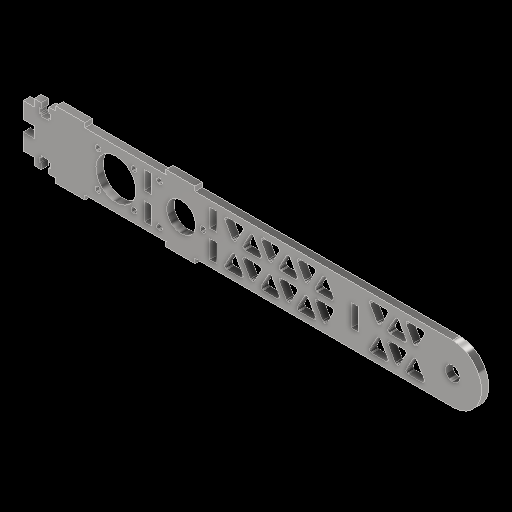
# Autodesk Inventor part: NeckFrame_Draft04
Saved by Autodesk Inventor 2022 (Build 260153000, 153)
## iProperties
Created: 2021-03-08
Part Number: NeckFrame_Draft04
Material: Steel, High Strength, Low Alloy
Document SubType Name: Modeling
Designer: M3rob
Density: 7.85 g/cm^3
Appearance: Steel - Polished
Mass: 5825.21 g
Surface Area: 1820.51 cm^2
Volume: 742.065 cm^3
Author: M3rob
Autodesk Inventor part; units mm, degrees
ref_plane "YZ Plane" through (0, 0, 0) normal (1, 0, 0) x (0, 1, 0)
ref_plane "XZ Plane" through (0, 0, 0) normal (0, 1, 0) x (-1, 0, 0)
ref_plane "XY Plane" through (0, 0, 0) normal (0, 0, 1) x (1, 0, 0)
sketch "Sketch1" plane through (0, 0, 0) normal (1, 0, 0) x (0, 1, 0)
  line L0 (50.8, 392.0089) -> (38.1, 392.0089)
  line L1 (-50.8, 392.0089) -> (-50.8, 366.2152)
  arc A0 (-50.8, -341.2089) -> (50.8, -341.2089) centre (0, -341.2089) ccw
  line L2 (50.8, -341.2089) -> (50.8, 110.0689)
  line L3 (50.8, -341.2089) -> (50.8, -392.0089) construction
  line L4 (50.8, -392.0089) -> (-50.8, -392.0089) construction
  line L5 (-50.8, -392.0089) -> (-50.8, -341.2089) construction
  line L6 (0, 392.0089) -> (0, -392.0089) construction
  line L7 (38.1, 392.0089) -> (38.1, 411.0589)
  line L8 (38.1, 411.0589) -> (9.525, 411.0589)
  line L9 (9.525, 411.0589) -> (9.525, 392.0089)
  line L10 (-9.525, 392.0089) -> (-9.525, 411.0589)
  line L11 (-9.525, 411.0589) -> (-38.1, 411.0589)
  line L12 (-38.1, 411.0589) -> (-38.1, 392.0089)
  line L13 (9.525, 392.0089) -> (-9.525, 392.0089)
  line L14 (38.1, 392.0089) -> (9.525, 392.0089) construction
  line L15 (-9.525, 392.0089) -> (-38.1, 392.0089) construction
  line L16 (-38.1, 392.0089) -> (-50.8, 392.0089)
  line L17 (39.6875, 84.6689) -> (7.9375, 84.6689)
  line L18 (7.9375, 84.6689) -> (7.9375, 71.9689)
  line L19 (7.9375, 71.9689) -> (39.6875, 71.9689)
  line L20 (39.6875, 71.9689) -> (39.6875, 84.6689)
  line L21 (39.6875, 84.6689) -> (7.9375, 71.9689) construction
  line L22 (7.9375, 84.6689) -> (39.6875, 71.9689) construction
  line L23 (-39.6875, 84.6689) -> (-7.9375, 84.6689)
  line L24 (-7.9375, 84.6689) -> (-7.9375, 71.9689)
  line L25 (-7.9375, 71.9689) -> (-39.6875, 71.9689)
  line L26 (-39.6875, 71.9689) -> (-39.6875, 84.6689)
  line L27 (-39.6875, 84.6689) -> (-7.9375, 71.9689) construction
  line L28 (-7.9375, 84.6689) -> (-39.6875, 71.9689) construction
  line L29 (50.8, 353.9089) -> (58.7375, 353.9089)
  line L30 (58.7375, 353.9089) -> (58.7375, 303.1089)
  line L31 (58.7375, 303.1089) -> (50.8, 303.1089)
  line L32 (50.8, 160.8689) -> (58.7375, 160.8689)
  line L33 (58.7375, 160.8689) -> (58.7375, 110.0689)
  line L34 (58.7375, 110.0689) -> (50.8, 110.0689)
  line L35 (-50.8, 110.0689) -> (-58.7375, 110.0689)
  line L36 (-58.7375, 110.0689) -> (-58.7375, 160.8689)
  line L37 (-58.7375, 160.8689) -> (-50.8, 160.8689)
  line L38 (7.9375, 198.9689) -> (39.6875, 198.9689)
  line L39 (39.6875, 198.9689) -> (39.6875, 186.2689)
  line L40 (39.6875, 186.2689) -> (7.9375, 186.2689)
  line L41 (7.9375, 186.2689) -> (7.9375, 198.9689)
  line L42 (7.9375, 198.9689) -> (39.6875, 186.2689) construction
  line L43 (39.6875, 198.9689) -> (7.9375, 186.2689) construction
  line L44 (-39.6875, 198.9689) -> (-7.9375, 198.9689)
  line L45 (-7.9375, 198.9689) -> (-7.9375, 186.2689)
  line L46 (-7.9375, 186.2689) -> (-39.6875, 186.2689)
  line L47 (-39.6875, 186.2689) -> (-39.6875, 198.9689)
  line L48 (-39.6875, 198.9689) -> (-7.9375, 186.2689) construction
  line L49 (-7.9375, 198.9689) -> (-39.6875, 186.2689) construction
  line L50 (23.8125, 192.6189) -> (23.8125, 78.3189) construction
  line L51 (-50.8, 353.9089) -> (-58.7375, 353.9089)
  line L52 (-58.7375, 353.9089) -> (-58.7375, 303.1089)
  line L53 (-58.7375, 303.1089) -> (-50.8, 303.1089)
  line L54 (50.8, 303.1089) -> (50.8, 353.9089) construction
  line L55 (50.8, 353.9089) -> (50.8, 392.0089) construction
  line L56 (-50.8, 303.1089) -> (-50.8, 353.9089) construction
  line L57 (-50.8, 353.9089) -> (-50.8, 303.1089) construction
  line L58 (-50.8, 160.8689) -> (-50.8, 110.0689) construction
  line L59 (-50.8, 110.0689) -> (-50.8, -341.2089)
  line L60 (50.8, 160.8689) -> (50.8, 303.1089)
  line L61 (50.8, 110.0689) -> (50.8, 160.8689) construction
  line L62 (50.8, 379.7026) -> (41.275, 379.7026)
  line L63 (41.275, 379.7026) -> (41.275, 382.4839)
  line L64 (41.275, 382.4839) -> (33.3375, 382.4839)
  line L65 (33.3375, 382.4839) -> (33.3375, 379.7026)
  line L66 (33.3375, 379.7026) -> (30.1625, 379.7026)
  line L67 (30.1625, 379.7026) -> (30.1625, 366.2152)
  line L68 (30.1625, 366.2152) -> (33.3375, 366.2152)
  line L69 (33.3375, 366.2152) -> (33.3375, 363.4339)
  line L70 (33.3375, 363.4339) -> (41.275, 363.4339)
  line L71 (41.275, 363.4339) -> (41.275, 366.2152)
  line L72 (41.275, 366.2152) -> (50.8, 366.2152)
  line L73 (30.1625, 372.9589) -> (50.8, 372.9589) construction
  line L74 (-50.8, 379.7026) -> (-41.275, 379.7026)
  line L75 (-41.275, 379.7026) -> (-41.275, 382.4839)
  line L76 (-41.275, 382.4839) -> (-33.3375, 382.4839)
  line L77 (-33.3375, 382.4839) -> (-33.3375, 379.7026)
  line L78 (-33.3375, 379.7026) -> (-30.1625, 379.7026)
  line L79 (-30.1625, 379.7026) -> (-30.1625, 366.2152)
  line L80 (-30.1625, 366.2152) -> (-33.3375, 366.2152)
  line L81 (-33.3375, 366.2152) -> (-33.3375, 363.4339)
  line L82 (-33.3375, 363.4339) -> (-41.275, 363.4339)
  line L83 (-41.275, 363.4339) -> (-41.275, 366.2152)
  line L84 (-50.8, 366.2152) -> (-41.275, 366.2152)
  line L85 (50.8, 379.7026) -> (50.8, 303.1089) construction
  line L86 (50.8, 366.2152) -> (50.8, 379.7026)
  line L87 (-50.8, 366.2152) -> (-50.8, 353.9089)
  line L88 (-50.8, 379.7026) -> (-50.8, 366.2152) construction
  circle A1 centre (0, 248.4989) radius 35.179
  circle A2 centre (0, 134.1989) radius 25.4
  line L89 (50.8, 379.7026) -> (50.8, 392.0089)
  line L90 (50.8, 366.2152) -> (50.8, 353.9089)
  circle A3 centre (0, -341.2089) radius 12.7
  line L91 (50.8, 353.9089) -> (50.8, 366.2152)
  line L92 (50.8, 303.1089) -> (50.8, 353.9089)
  line L93 (-50.8, 353.9089) -> (-50.8, 379.7026)
  line L94 (-50.8, 303.1089) -> (-50.8, 160.8689)
  line L95 (-50.8, 353.9089) -> (-50.8, 303.1089) construction
  line L96 (-50.8, 366.2152) -> (-50.8, 353.9089)
  circle A4 centre (0, 248.4989) radius 44.45 construction
  circle A5 centre (31.4309, 279.9298) radius 5.08 construction
  line L97 (31.4309, 279.9298) -> (0, 248.4989) construction
  circle A6 centre (-31.4309, 279.9298) radius 5.08 construction
  circle A7 centre (-31.4309, 217.068) radius 5.08 construction
  circle A8 centre (31.4309, 217.068) radius 5.08 construction
  circle A9 centre (34.925, 172.2989) radius 5.08 construction
  circle A10 centre (-34.925, 172.2989) radius 5.08 construction
  circle A11 centre (0, 96.0989) radius 5.08 construction
  line L98 (19.05, -163.6161) -> (-19.05, -163.6161)
  line L99 (-19.05, -163.6161) -> (-19.05, -176.3161)
  line L100 (-19.05, -176.3161) -> (19.05, -176.3161)
  line L101 (19.05, -176.3161) -> (19.05, -163.6161)
  point P0 (0, 0)
  point P1 (-23.8125, 78.3189)
  point P2 (23.8125, 192.6189)
  point P3 (-23.8125, 192.6189)
  point P4 (23.8125, 411.0589)
  point P5 (58.7375, 135.4689)
  point P6 (23.8125, 135.4689)
  point P7 (23.8125, 372.9589)
  point P8 (-30.1625, 372.9589)
  point P9 (50.8, 353.9089)
  point P10 (50.8, 303.1089)
  point P11 (-50.8, 379.7026)
  point P12 (-50.8, 366.2152)
  point P13 (-50.8, 353.9089)
  point P14 (-50.8, 353.9089)
  point P15 (-50.8, 303.1089)
  point P16 (0, -378.889)
  point P17 (0, 0)
  point P18 (0, -163.6161)
  dimension "d130" = 88.9
  dimension "d0" = 101.6
  dimension "d3" = 19.05
  dimension "d4" = 12.7
  dimension "d5" = 19.05
  dimension "d6" = 12.7
  dimension "d8" = 7.9375
  dimension "d9" = 50.8
  dimension "d12" = 31.75
  dimension "d13" = 38.1
  dimension "d14" = 9.525
  dimension "d15" = 7.9375
  dimension "d16" = 3.175
  dimension "d17" = 19.05
  dimension "d18" = 13.4874
  dimension "d23" = 143.51
  dimension "d24" = 70.358
  dimension "d25" = 50.8
  dimension "d26" = 19.05
  dimension "d39" = 25.4
  dimension "d86" = 101.6
  dimension "d92" = 193.04
  dimension "d98" = 7.9375
  dimension "d99" = 0
  dimension "d100" = 7.9375
  dimension "d101" = 50.8
  dimension "d102" = 34.925
  dimension "d104" = 732.7979
  dimension "d105" = 109.5375
  dimension "d106" = 25.7937
  dimension "d107" = 109.5375
  dimension "d108" = 12.3063
  dimension "d109" = 109.5375
  dimension "d110" = 0
  dimension "d111" = 109.5375
  dimension "d112" = 0
  dimension "d113" = 109.5375
  dimension "d114" = 50.8
  dimension "d116" = 45
  dimension "d118" = 10.16
  dimension "d121" = 360
  dimension "d131" = 114.3
  dimension "d132" = 475.4078
  dimension "d135" = 10.16
  dimension "d136" = 38.1
  dimension "d138" = 38.1
  dimension "d139" = 69.85
  dimension "d161" = 555.625
  dimension "d162" = 12.7
  dimension "d163" = 38.1
  constraints: 204 end point, 125 perpendicular, 34 point on line, 21 tangent, 19 midpoint, 15 equal length, 15 horizontal, 14 vertical, 11 centre point, 11 parallel, 6 horizontal alignment, 3 collinear, 3 vertical alignment, 2 coincident, 2 equal radius, 2 point on circle, 1 concentric, 1 symmetric about line, 18 other
  measures "d0" distance of L0.start L1.start
  measures "d3" diameter of L9 L6
  measures "d4" distance from line of L0.start L7
  measures "d5" distance of L0.end L7.end
  measures "d6" distance of L19.end L17.start
  measures "d8" distance of L33.end L2.end
  measures "d9" distance of L32.end L33.end
  measures "d12" distance of L18.end L19.end
  measures "d13" distance from line of L29 L0.start
  measures "d14" distance of L71.end L72.end
  measures "d15" distance of L69.end L70.end
  measures "d16" distance of L67.end L68.end
  measures "d17" distance of L69.end L64.end
  measures "d18" distance between parallel lines of L72 L62
  measures "d23" distance from line of L14 A1.centre
  measures "d24" diameter of A1
  measures "d25" diameter of A2
  measures "d26" distance from line of L0 L73.end
  measures "d39" diameter of A3
  measures "d86" distance between parallel lines of L40 L17
  measures "d92" distance between parallel lines of L38 L0
  measures "d98" distance from line of point (50.8, 353.909) L30
  measures "d99" distance from line of point (50.8, 353.909) L29
  measures "d100" distance from line of point (50.8, 303.109) L30
  measures "d101" distance from line of point (50.8, 303.109) L29
  measures "d102" distance from line of point (23.812, 372.959) L30
  measures "d104" distance from line of point (0, -378.889) L29
  measures "d105" distance from line of point (-50.8, 379.703) L30
  measures "d106" distance from line of point (-50.8, 379.703) L29
  measures "d107" distance from line of point (-50.8, 366.215) L30
  measures "d108" distance from line of point (-50.8, 366.215) L29
  measures "d109" distance from line of point (-50.8, 353.909) L30
  measures "d110" distance from line of point (-50.8, 353.909) L29
  measures "d111" distance from line of point (-50.8, 353.909) L30
  measures "d112" distance from line of point (-50.8, 353.909) L29
  measures "d113" distance from line of point (-50.8, 303.109) L30
  measures "d114" distance from line of point (-50.8, 303.109) L29
  measures "d116" angle of L6 L97
  measures "d118" diameter of A5
  measures "d131" distance of A2.centre A1.centre
  measures "d132" distance of A0.centre A2.centre
  measures "d135" diameter of A9
  measures "d136" vertical distance of A2.centre A9.centre
  measures "d138" distance of A11.centre A2.centre
  measures "d139" diameter of A9.centre L6
  measures "d161" distance between parallel lines of L98 L13
  measures "d162" distance between parallel lines of L100 L98
  measures "d163" distance of L98.start L98.end
extrude "Extrusion1" add sketch "Sketch1" along normal mid plane 12.7 contours L89 L62 L63 L64 L65 L66 L67 L68 L69 L70 L71 L72 L90 L92 L60 L32 L33 L34 L2 A0 L59 L35 L36 L37 L94 L53 L52 L51 L87 L84 L83 L82 L81 L80 L79 L78 L77 L76 L75 L74 L1 L16 L12 L11 L10 L13 L9 L8 L7 L0 | L29 L30 L31 L92
sketch "Sketch6" plane through (6.35, 0, 0) normal (1, 0, 0) x (0, 0, -1)
  point P0 (0, 0)
  point P1 (-279.9298, 31.4309)
  point P2 (-279.9298, -31.4309)
  point P3 (-217.068, -31.4309)
  point P4 (-217.068, 31.4309)
  point P5 (-172.2989, 34.925)
  point P6 (-172.2989, -34.925)
  point P7 (-96.0989, 0)
hole "Hole2" at (6.35, 31.4309, 279.9298) at (6.35, -31.4309, 279.9298) at (6.35, -31.4309, 217.068) at (6.35, 31.4309, 217.068) at (6.35, 34.925, 172.2989) at (6.35, -34.925, 172.2989) at (6.35, 0, 96.0989) direction (-1, 0, 0) diameter 10.0838 end through all clearance for "Flat Head Machine Screw (82)" size "3/8" standard "Ansi Unified Screw Threads"
sketch "Sketch7" plane through (6.35, 0, 0) normal (1, 0, 0) x (0, 0, -1)
  line L0 (-57.5666, 33.7863) -> (-45.2955, 11.7744)
  line L1 (-38.3626, 11.7744) -> (-26.0915, 33.7863)
  line L2 (-29.5579, 39.6875) -> (-54.1001, 39.6875)
  line L3 (-13.5455, 33.4693) -> (-25.8166, 11.4575)
  line L4 (-22.3501, 5.5563) -> (2.1921, 5.5563)
  line L5 (5.6585, 11.4575) -> (-6.6126, 33.4693)
  circle A0 centre (341.2089, 0) radius 12.7 projected
  line L6 (341.2089, 0) -> (-392.0089, 0) construction
  line L7 (-392.0089, -9.525) -> (-392.0089, 9.525) projected
  arc A1 (-54.1001, 39.6875) -> (-57.5666, 33.7863) centre (-54.1001, 35.7187) ccw
  arc A2 (-26.0915, 33.7863) -> (-29.5579, 39.6875) centre (-29.5579, 35.7187) ccw
  arc A3 (-45.2955, 11.7744) -> (-38.3626, 11.7744) centre (-41.829, 13.7069) ccw
  arc A4 (-25.8166, 11.4575) -> (-22.3501, 5.5563) centre (-22.3501, 9.525) ccw
  arc A5 (-6.6126, 33.4693) -> (-13.5455, 33.4693) centre (-10.079, 31.5369) ccw
  arc A6 (2.1921, 5.5563) -> (5.6585, 11.4575) centre (2.1921, 9.525) ccw
  line L8 (-57.5666, -33.7863) -> (-45.2955, -11.7744)
  line L9 (-38.3626, -11.7744) -> (-26.0915, -33.7863)
  line L10 (-29.5579, -39.6875) -> (-54.1001, -39.6875)
  line L11 (-13.5455, -33.4693) -> (-25.8166, -11.4575)
  line L12 (-22.3501, -5.5563) -> (2.1921, -5.5563)
  line L13 (5.6585, -11.4575) -> (-6.6126, -33.4693)
  arc A7 (-57.5666, -33.7863) -> (-54.1001, -39.6875) centre (-54.1001, -35.7187) ccw
  arc A8 (-29.5579, -39.6875) -> (-26.0915, -33.7863) centre (-29.5579, -35.7187) ccw
  arc A9 (-38.3626, -11.7744) -> (-45.2955, -11.7744) centre (-41.829, -13.7069) ccw
  arc A10 (-22.3501, -5.5563) -> (-25.8166, -11.4575) centre (-22.3501, -9.525) ccw
  arc A11 (-13.5455, -33.4693) -> (-6.6126, -33.4693) centre (-10.079, -31.5369) ccw
  arc A12 (5.6585, -11.4575) -> (2.1921, -5.5563) centre (2.1921, -9.525) ccw
  arc A13 (37.4085, 33.7863) -> (33.9421, 39.6875) centre (33.9421, 35.7187) ccw
  line L14 (25.1374, 11.7744) -> (37.4085, 33.7863)
  line L15 (5.9334, 33.7863) -> (18.2045, 11.7744)
  line L16 (33.9421, 39.6875) -> (9.3999, 39.6875)
  arc A14 (9.3999, 39.6875) -> (5.9334, 33.7863) centre (9.3999, 35.7187) ccw
  arc A15 (37.6834, 11.4575) -> (41.1499, 5.5563) centre (41.1499, 9.525) ccw
  line L17 (49.9545, 33.4693) -> (37.6834, 11.4575)
  arc A16 (56.8874, 33.4693) -> (49.9545, 33.4693) centre (53.421, 31.5369) ccw
  line L18 (69.1585, 11.4575) -> (56.8874, 33.4693)
  line L19 (41.1499, 5.5563) -> (65.6921, 5.5563)
  arc A17 (65.6921, 5.5563) -> (69.1585, 11.4575) centre (65.6921, 9.525) ccw
  line L20 (41.1499, -5.5563) -> (65.6921, -5.5563)
  arc A18 (41.1499, -5.5563) -> (37.6834, -11.4575) centre (41.1499, -9.525) ccw
  arc A19 (69.1585, -11.4575) -> (65.6921, -5.5563) centre (65.6921, -9.525) ccw
  line L21 (49.9545, -33.4693) -> (37.6834, -11.4575)
  line L22 (69.1585, -11.4575) -> (56.8874, -33.4693)
  arc A20 (49.9545, -33.4693) -> (56.8874, -33.4693) centre (53.421, -31.5369) ccw
  arc A21 (18.2045, 11.7744) -> (25.1374, 11.7744) centre (21.671, 13.7069) ccw
  arc A22 (33.9421, -39.6875) -> (37.4085, -33.7863) centre (33.9421, -35.7187) ccw
  line L23 (25.1374, -11.7744) -> (37.4085, -33.7863)
  arc A23 (25.1374, -11.7744) -> (18.2045, -11.7744) centre (21.671, -13.7069) ccw
  line L24 (33.9421, -39.6875) -> (9.3999, -39.6875)
  line L25 (5.9334, -33.7863) -> (18.2045, -11.7744)
  arc A24 (5.9334, -33.7863) -> (9.3999, -39.6875) centre (9.3999, -35.7187) ccw
  arc A25 (100.9085, 33.7863) -> (97.4421, 39.6875) centre (97.4421, 35.7187) ccw
  line L26 (88.6374, 11.7744) -> (100.9085, 33.7863)
  line L27 (69.4334, 33.7863) -> (81.7045, 11.7744)
  line L28 (97.4421, 39.6875) -> (72.8999, 39.6875)
  arc A26 (72.8999, 39.6875) -> (69.4334, 33.7863) centre (72.8999, 35.7187) ccw
  arc A27 (101.1834, 11.4575) -> (104.6499, 5.5563) centre (104.6499, 9.525) ccw
  line L29 (113.4545, 33.4693) -> (101.1834, 11.4575)
  arc A28 (120.3874, 33.4693) -> (113.4545, 33.4693) centre (116.921, 31.5369) ccw
  line L30 (132.6585, 11.4575) -> (120.3874, 33.4693)
  line L31 (104.6499, 5.5563) -> (129.1921, 5.5563)
  arc A29 (129.1921, 5.5563) -> (132.6585, 11.4575) centre (129.1921, 9.525) ccw
  line L32 (104.6499, -5.5563) -> (129.1921, -5.5563)
  arc A30 (104.6499, -5.5563) -> (101.1834, -11.4575) centre (104.6499, -9.525) ccw
  arc A31 (132.6585, -11.4575) -> (129.1921, -5.5563) centre (129.1921, -9.525) ccw
  line L33 (113.4545, -33.4693) -> (101.1834, -11.4575)
  line L34 (132.6585, -11.4575) -> (120.3874, -33.4693)
  arc A32 (113.4545, -33.4693) -> (120.3874, -33.4693) centre (116.921, -31.5369) ccw
  arc A33 (81.7045, 11.7744) -> (88.6374, 11.7744) centre (85.171, 13.7069) ccw
  arc A34 (97.4421, -39.6875) -> (100.9085, -33.7863) centre (97.4421, -35.7187) ccw
  line L35 (88.6374, -11.7744) -> (100.9085, -33.7863)
  arc A35 (88.6374, -11.7744) -> (81.7045, -11.7744) centre (85.171, -13.7069) ccw
  line L36 (97.4421, -39.6875) -> (72.8999, -39.6875)
  line L37 (69.4334, -33.7863) -> (81.7045, -11.7744)
  arc A36 (69.4334, -33.7863) -> (72.8999, -39.6875) centre (72.8999, -35.7187) ccw
  arc A37 (164.4085, 33.7863) -> (160.9421, 39.6875) centre (160.9421, 35.7187) ccw
  line L38 (152.1374, 11.7744) -> (164.4085, 33.7863)
  line L39 (132.9334, 33.7863) -> (145.2045, 11.7744)
  line L40 (160.9421, 39.6875) -> (136.3999, 39.6875)
  arc A38 (136.3999, 39.6875) -> (132.9334, 33.7863) centre (136.3999, 35.7187) ccw
  arc A39 (164.6834, 11.4575) -> (168.1499, 5.5563) centre (168.1499, 9.525) ccw
  line L41 (176.9545, 33.4693) -> (164.6834, 11.4575)
  arc A40 (183.8874, 33.4693) -> (176.9545, 33.4693) centre (180.421, 31.5369) ccw
  line L42 (196.1585, 11.4575) -> (183.8874, 33.4693)
  line L43 (168.1499, 5.5563) -> (192.6921, 5.5563)
  arc A41 (192.6921, 5.5563) -> (196.1585, 11.4575) centre (192.6921, 9.525) ccw
  line L44 (168.1499, -5.5563) -> (192.6921, -5.5563)
  arc A42 (168.1499, -5.5563) -> (164.6834, -11.4575) centre (168.1499, -9.525) ccw
  arc A43 (196.1585, -11.4575) -> (192.6921, -5.5563) centre (192.6921, -9.525) ccw
  line L45 (176.9545, -33.4693) -> (164.6834, -11.4575)
  line L46 (196.1585, -11.4575) -> (183.8874, -33.4693)
  arc A44 (176.9545, -33.4693) -> (183.8874, -33.4693) centre (180.421, -31.5369) ccw
  arc A45 (145.2045, 11.7744) -> (152.1374, 11.7744) centre (148.671, 13.7069) ccw
  arc A46 (160.9421, -39.6875) -> (164.4085, -33.7863) centre (160.9421, -35.7187) ccw
  line L47 (152.1374, -11.7744) -> (164.4085, -33.7863)
  arc A47 (152.1374, -11.7744) -> (145.2045, -11.7744) centre (148.671, -13.7069) ccw
  line L48 (160.9421, -39.6875) -> (136.3999, -39.6875)
  line L49 (132.9334, -33.7863) -> (145.2045, -11.7744)
  arc A48 (132.9334, -33.7863) -> (136.3999, -39.6875) centre (136.3999, -35.7187) ccw
  arc A49 (227.9085, 33.7863) -> (224.4421, 39.6875) centre (224.4421, 35.7187) ccw
  line L50 (215.6374, 11.7744) -> (227.9085, 33.7863)
  line L51 (196.4334, 33.7863) -> (208.7045, 11.7744)
  line L52 (224.4421, 39.6875) -> (199.8999, 39.6875)
  arc A50 (199.8999, 39.6875) -> (196.4334, 33.7863) centre (199.8999, 35.7187) ccw
  arc A51 (228.1834, 11.4575) -> (231.6499, 5.5563) centre (231.6499, 9.525) ccw
  line L53 (240.4545, 33.4693) -> (228.1834, 11.4575)
  arc A52 (247.3874, 33.4693) -> (240.4545, 33.4693) centre (243.921, 31.5369) ccw
  line L54 (259.6585, 11.4575) -> (247.3874, 33.4693)
  line L55 (231.6499, 5.5563) -> (256.1921, 5.5563)
  arc A53 (256.1921, 5.5563) -> (259.6585, 11.4575) centre (256.1921, 9.525) ccw
  line L56 (231.6499, -5.5563) -> (256.1921, -5.5563)
  arc A54 (231.6499, -5.5563) -> (228.1834, -11.4575) centre (231.6499, -9.525) ccw
  arc A55 (259.6585, -11.4575) -> (256.1921, -5.5563) centre (256.1921, -9.525) ccw
  line L57 (240.4545, -33.4693) -> (228.1834, -11.4575)
  line L58 (259.6585, -11.4575) -> (247.3874, -33.4693)
  arc A56 (240.4545, -33.4693) -> (247.3874, -33.4693) centre (243.921, -31.5369) ccw
  arc A57 (208.7045, 11.7744) -> (215.6374, 11.7744) centre (212.171, 13.7069) ccw
  arc A58 (224.4421, -39.6875) -> (227.9085, -33.7863) centre (224.4421, -35.7187) ccw
  line L59 (215.6374, -11.7744) -> (227.9085, -33.7863)
  arc A59 (215.6374, -11.7744) -> (208.7045, -11.7744) centre (212.171, -13.7069) ccw
  line L60 (224.4421, -39.6875) -> (199.8999, -39.6875)
  line L61 (196.4334, -33.7863) -> (208.7045, -11.7744)
  arc A60 (196.4334, -33.7863) -> (199.8999, -39.6875) centre (199.8999, -35.7187) ccw
  arc A61 (291.4085, 33.7863) -> (287.9421, 39.6875) centre (287.9421, 35.7187) ccw
  line L62 (279.1374, 11.7744) -> (291.4085, 33.7863)
  line L63 (259.9334, 33.7863) -> (272.2045, 11.7744)
  line L64 (287.9421, 39.6875) -> (263.3999, 39.6875)
  arc A62 (263.3999, 39.6875) -> (259.9334, 33.7863) centre (263.3999, 35.7187) ccw
  arc A63 (291.6834, 11.4575) -> (295.1499, 5.5563) centre (295.1499, 9.525) ccw
  line L65 (303.9545, 33.4693) -> (291.6834, 11.4575)
  arc A64 (310.8874, 33.4693) -> (303.9545, 33.4693) centre (307.421, 31.5369) ccw
  line L66 (323.1585, 11.4575) -> (310.8874, 33.4693)
  line L67 (295.1499, 5.5563) -> (319.6921, 5.5563)
  arc A65 (319.6921, 5.5563) -> (323.1585, 11.4575) centre (319.6921, 9.525) ccw
  line L68 (295.1499, -5.5563) -> (319.6921, -5.5563)
  arc A66 (295.1499, -5.5563) -> (291.6834, -11.4575) centre (295.1499, -9.525) ccw
  arc A67 (323.1585, -11.4575) -> (319.6921, -5.5563) centre (319.6921, -9.525) ccw
  line L69 (303.9545, -33.4693) -> (291.6834, -11.4575)
  line L70 (323.1585, -11.4575) -> (310.8874, -33.4693)
  arc A68 (303.9545, -33.4693) -> (310.8874, -33.4693) centre (307.421, -31.5369) ccw
  arc A69 (272.2045, 11.7744) -> (279.1374, 11.7744) centre (275.671, 13.7069) ccw
  arc A70 (287.9421, -39.6875) -> (291.4085, -33.7863) centre (287.9421, -35.7187) ccw
  line L71 (279.1374, -11.7744) -> (291.4085, -33.7863)
  arc A71 (279.1374, -11.7744) -> (272.2045, -11.7744) centre (275.671, -13.7069) ccw
  line L72 (287.9421, -39.6875) -> (263.3999, -39.6875)
  line L73 (259.9334, -33.7863) -> (272.2045, -11.7744)
  arc A72 (259.9334, -33.7863) -> (263.3999, -39.6875) centre (263.3999, -35.7187) ccw
  point P0 (0, 0)
  point P1 (-60.8564, 39.6875)
  point P2 (-41.829, 5.5563)
  point P3 (-22.8017, 39.6875)
  point P4 (-10.079, 39.6875)
  point P5 (-71.9689, 39.6875)
  point P6 (-41.829, 39.6875)
  point P7 (-60.8564, -39.6875)
  point P8 (-41.829, -5.5563)
  point P9 (-22.8017, -39.6875)
  point P10 (-10.079, -39.6875)
  point P11 (-41.829, -39.6875)
  point P12 (21.671, 5.5563)
  point P13 (40.6983, 39.6875)
  point P14 (21.671, 39.6875)
  point P15 (2.6436, 39.6875)
  point P16 (53.421, 39.6875)
  point P17 (53.421, -39.6875)
  point P18 (40.6983, -39.6875)
  point P19 (21.671, -5.5563)
  point P20 (21.671, -39.6875)
  point P21 (2.6436, -39.6875)
  point P22 (85.171, 5.5563)
  point P23 (104.1983, 39.6875)
  point P24 (85.171, 39.6875)
  point P25 (66.1436, 39.6875)
  point P26 (116.921, 39.6875)
  point P27 (116.921, -39.6875)
  point P28 (104.1983, -39.6875)
  point P29 (85.171, -5.5563)
  point P30 (85.171, -39.6875)
  point P31 (66.1436, -39.6875)
  point P32 (148.671, 5.5563)
  point P33 (167.6983, 39.6875)
  point P34 (148.671, 39.6875)
  point P35 (129.6436, 39.6875)
  point P36 (180.421, 39.6875)
  point P37 (180.421, -39.6875)
  point P38 (167.6983, -39.6875)
  point P39 (148.671, -5.5563)
  point P40 (148.671, -39.6875)
  point P41 (129.6436, -39.6875)
  point P42 (212.171, 5.5563)
  point P43 (231.1983, 39.6875)
  point P44 (212.171, 39.6875)
  point P45 (193.1436, 39.6875)
  point P46 (243.921, 39.6875)
  point P47 (243.921, -39.6875)
  point P48 (231.1983, -39.6875)
  point P49 (212.171, -5.5563)
  point P50 (212.171, -39.6875)
  point P51 (193.1436, -39.6875)
  point P52 (275.671, 5.5563)
  point P53 (294.6983, 39.6875)
  point P54 (275.671, 39.6875)
  point P55 (256.6436, 39.6875)
  point P56 (307.421, 39.6875)
  point P57 (307.421, -39.6875)
  point P58 (294.6983, -39.6875)
  point P59 (275.671, -5.5563)
  point P60 (275.671, -39.6875)
  point P61 (256.6436, -39.6875)
  dimension "d141" = 11.1125
  dimension "d142" = 11.1125
  dimension "d144" = 11.1125
  dimension "d147" = 3.9688
  dimension "d148" = 3.9688
  dimension "d149" = 31.75
  dimension "d152" = 63.5
  constraints: 146 end point, 144 point on circle, 96 point on line, 72 centre point, 23 symmetric about line, 12 tangent, 4 equal radius, 2 equal length, 2 horizontal, 2 horizontal alignment, 2 midpoint, 2 parallel, 1 vertical alignment, 356 other
  measures "d141" diameter of L4 L6
  measures "d142" distance of point (-71.969, 39.687) point (-60.856, 39.687)
  measures "d144" distance between parallel lines of L1 L3
  measures "d147" radius of A1
  measures "d148" radius of A2
  measures "d149" horizontal distance of point (-41.829, 5.556) point (-10.079, 39.687)
  measures "d152" distance of L1.end L14.end
extrude "Extrusion4" cut sketch "Sketch7" against normal through all contours A1 L2 A2 L1 A3 L0 | A5 L5 A6 L4 A4 L3 | L8 A9 L9 A8 L10 A7 | L11 A10 L12 A12 L13 A11 | L14 A21 L15 A14 L16 A13 | L17 A16 L18 A17 L19 A15 | L20 A19 L22 A20 L21 A18 | L24 A24 L25 A23 L23 A22 | L26 A33 L27 A26 L28 A25 | L29 A28 L30 A29 L31 A27 | L32 A31 L34 A32 L33 A30 | L36 A36 L37 A35 L35 A34 | L50 A57 L51 A50 L52 A49 | L53 A52 L54 A53 L55 A51 | L56 A55 L58 A56 L57 A54 | L60 A60 L61 A59 L59 A58 | L62 A69 L63 A62 L64 A61 | L72 A72 L73 A71 L71 A70
equation "\"d26\" = 0.5 * d13"
body "Solid1"
